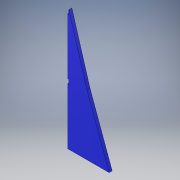
# Autodesk Inventor part: Fin
Saved by Autodesk Inventor 2018 (Build 220112000, 112)
## iProperties
Created: 2017-10-02
Part Number: Fin
Material: Generic
Document SubType Name: Modeling
Designer: Intel
Density: 1 g/cm^3
Appearance: Blue - Wall Paint - Glossy
Author: Intel
Autodesk Inventor part; units mm, degrees
ref_plane "YZ Plane" through (0, 0, 0) normal (1, 0, 0) x (0, 1, 0)
ref_plane "XZ Plane" through (0, 0, 0) normal (0, 1, 0) x (-1, 0, 0)
ref_plane "XY Plane" through (0, 0, 0) normal (0, 0, 1) x (1, 0, 0)
sketch "Sketch1" plane through (0, 0, 0) normal (0, 0, 1) x (1, 0, 0)
  line L0 (-63.5, -190.5) -> (63.5, -190.5)
  line L1 (63.5, -190.5) -> (63.5, 190.5) construction
  line L2 (63.5, 190.5) -> (-63.5, 190.5) construction
  line L3 (-63.5, 190.5) -> (-63.5, -190.5)
  line L4 (-63.5, -190.5) -> (63.5, 190.5) construction
  line L5 (63.5, -190.5) -> (-63.5, 190.5) construction
  line L6 (-63.5, 190.5) -> (-6.35, 0)
  line L7 (-6.35, 0) -> (63.5, -190.5)
  line L8 (-63.5, -190.5) -> (-66.675, -190.5)
  line L9 (-66.675, -190.5) -> (-66.675, -12.7)
  line L10 (-66.675, -12.7) -> (-63.5, -12.7)
  line L11 (-63.5, -12.7) -> (-63.5, -190.5)
  line L12 (-63.5, 0) -> (-66.675, 0)
  line L13 (-66.675, 0) -> (-66.675, 177.8)
  line L14 (-66.675, 177.8) -> (-63.5, 177.8)
  line L15 (-63.5, 177.8) -> (-63.5, 0)
  point P0 (0, 0)
  dimension "d0" = 381
  dimension "d1" = 127
  dimension "d2" = 190.5
  dimension "d3" = 57.15
  dimension "d7" = 3.175
  dimension "d8" = 177.8
  dimension "d9" = 3.175
  dimension "d10" = 12.7
  dimension "d11" = 12.7
  constraints: 32 end point, 6 parallel, 3 horizontal, 3 midpoint, 3 perpendicular
  measures "d0" distance of L1.end L0.end
  measures "d1" distance of L0.start L0.end
  measures "d2" distance from line of L0 L6.end
  measures "d3" distance from line of L3 L6.end
  measures "d7" distance between parallel lines of L3 L9
  measures "d8" distance between parallel lines of L0 L10
  measures "d9" distance of L13.end L14.end
  measures "d10" distance between parallel lines of L12 L10
  measures "d11" distance from line of L2.end L14
extrude "Extrusion1" add sketch "Sketch1" along normal blind 9.525
equation "\"d2\" = 0.5 * d0"
body "Solid1"
